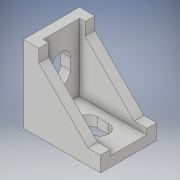
# Autodesk Inventor part: bracket
Saved by Autodesk Inventor 2019.3 (Build 233278000, 278)
## iProperties
Created: 2019-04-14
Part Number: bracket
Material: Generic
Document SubType Name: Modeling
Designer: peter
Density: 1 g/cm^3
Appearance: Default
Author: peter
Autodesk Inventor part; units mm, degrees
ref_plane "YZ Plane" through (0, 0, 0) normal (1, 0, 0) x (0, 1, 0)
sketch "Sketch1" plane through (0, 0, 0) normal (0, 0, 1) x (1, 0, 0)
  line L0 (0, 0) -> (27.5, 0)
  line L1 (27.5, 0) -> (27.5, 5.5)
  line L2 (27.5, 5.5) -> (23, 5.5)
  line L3 (0, 0) -> (0, 27.5)
  line L4 (0, 0) -> (27.5, 0) construction
  line L5 (0, 27.5) -> (5.5, 27.5)
  line L6 (5.5, 27.5) -> (5.5, 23)
  line L7 (5.5, 23) -> (23, 5.5)
  dimension "d0" = 27.5
  dimension "d1" = 5.5
  dimension "d2" = 4.5
  dimension "d3" = 27.5
  dimension "d4" = 90
  dimension "d5" = 5.5
  dimension "d6" = 4.5
  constraints: 16 end point, 5 perpendicular, 2 horizontal, 1 vertical
  measures "d0" distance of L0.start L0.end
  measures "d1" distance of L0.end L1.end
  measures "d2" distance of L1.end L2.end
  measures "d3" distance of L0.start L3.end
  measures "d4" angle of L4 L3
  measures "d5" distance of L3.end L5.end
  measures "d6" distance of L5.end L6.end
sketch "Sketch2" plane through (0, 0, 0) normal (0, 0, 1) x (1, 0, 0)
  line L0 (0, 0) -> (3.5, 0)
  line L1 (3.5, 3.5) -> (3.5, 27.5)
  line L2 (3.5, 27.5) -> (0, 27.5)
  line L3 (0, 27.5) -> (0, 0)
  line L4 (0, 0) -> (27.5, 0)
  line L5 (27.5, 0) -> (27.5, 3.5)
  line L6 (27.5, 3.5) -> (3.5, 3.5)
  line L7 (0, 3.5) -> (0, 0)
  dimension "d7" = 3.5
  dimension "d8" = 27.5
  dimension "d9" = 27.5
  dimension "d10" = 3.5
  constraints: 16 end point, 4 parallel, 2 horizontal, 2 perpendicular
  measures "d7" distance of L2.end L1.end
  measures "d8" distance of L1.end L0.end
  measures "d9" distance of L7.start L5.end
  measures "d10" distance of L5.end L4.end
extrude "Extrusion1" add sketch "Sketch2" against normal blind 20
extrude "Extrusion2" add sketch "Sketch1" against normal blind 3.5
ref_plane "Work Plane1" through (0, 0, -10) normal (0, 0, 1) x (1, 0, 0)
mirror "Mirror1" about plane through (0, 0, -10) normal (0, 0, 1) of "Extrusion2"
sketch "Sketch3" plane through (0, 0, 0) normal (-1, 0, 0) x (0, 0, 1)
  line L0 (0, 0) -> (-20, 0) construction
  line L1 (-10, 0) -> (-10, 15) construction
  line L2 (-10, 14.8275) -> (-6.75, 14.8275) construction
  line L3 (-6.75, 14.8275) -> (-6.75, 9.8275) construction
  line L4 (-10, 9.8275) -> (-10, 14.8275) construction
  line L5 (-13.25, 13.0775) -> (-13.25, 17.1562)
  line L6 (-10, 20.4062) -> (-10, 20.4062)
  line L7 (-6.75, 17.1562) -> (-6.75, 13.0775)
  arc A0 (-10, 20.4062) -> (-13.25, 17.1562) centre (-10, 17.1562) ccw
  arc A1 (-6.75, 17.1562) -> (-10, 20.4062) centre (-10, 17.1562) ccw
  arc A2 (-13.25, 13.0775) -> (-10, 9.8275) centre (-10, 13.0775) ccw
  line L8 (-10, 9.8275) -> (-10, 9.8275)
  arc A3 (-10, 9.8275) -> (-6.75, 13.0775) centre (-10, 13.0775) ccw
  point P0 (-13.25, 20.4062)
  point P1 (-6.75, 20.4062)
  dimension "d16" = 15
  dimension "d17" = 3.25
  dimension "d18" = 5
  dimension "d19" = 6.5
  dimension "d20" = 3.25
  dimension "d21" = 3.25
  constraints: 16 end point, 8 point on circle, 7 point on line, 7 tangent, 4 centre point, 2 equal radius, 2 horizontal, 2 parallel, 1 midpoint, 1 perpendicular, 1 vertical
  measures "d16" distance of L1.start L1.end
  measures "d17" distance of L3.end L4.start
  measures "d18" distance of L2.end L3.end
  measures "d19" distance of point (-13.25, 20.406) point (-6.75, 20.406)
  measures "d20" radius of A0
  measures "d21" radius of A3
extrude "Extrusion3" cut sketch "Sketch3" against normal through all
ref_plane "Work Plane2" through (0, 0, 0) normal (0.7071, -0.7071, 0) x (0, 0, -1)
mirror "Mirror2" about plane through (0, 0, 0) normal (0.7071, -0.7071, 0) of "Extrusion3"
body "Solid1"
